Make one of these (Autodesk Fusion 360 design; units mm, degrees)
Autodesk Fusion 360 part; units mm, degrees
sketch "Sketch1" plane through (0, 0, 0) normal (0, 1, 0) x (1, 0, 0)
  line L0 (0, 0) -> (76.2, 0)
  line L1 (76.2, 0) -> (76.2, 266.7)
  line L2 (76.2, 266.7) -> (0, 266.7)
  line L3 (0, 266.7) -> (0, 0)
  constraint horizontal L0
  constraint vertical L1
  constraint horizontal L2
  constraint vertical L3
  constraint coincident L0.start L3.end
extrude "Extrude1" add sketch "Sketch1" along normal blind 6.35
sketch "Sketch2" plane through (0, 6.35, 0) normal (0, 1, 0) x (-1, 0, 0)
  line L0 (0, -266.7) -> (0, 0)
  line L1 (0, 0) -> (-76.2, 0)
  line L2 (-76.2, 0) -> (-76.2, -266.7)
  line L3 (-76.2, -266.7) -> (0, -266.7)
  circle A0 centre (-25.4, -12.7) radius 1.27
  dimension "d3" = 2.54
  measures "d3" diameter of A0
extrude "Extrude2" cut sketch "Sketch2" against normal blind 6.35 contours A0
sketch "Sketch3" plane through (0, 6.35, 0) normal (0, 1, 0) x (-1, 0, 0)
  circle A0 centre (-25.4, -12.7) radius 1.27
  line L0 (0, -266.7) -> (0, 0)
  line L1 (0, 0) -> (-76.2, 0)
  line L2 (-76.2, 0) -> (-76.2, -266.7)
  line L3 (-76.2, -266.7) -> (0, -266.7)
  circle A1 centre (-50.8, -12.7) radius 1.27
  circle A2 centre (-25.4, -254) radius 1.27
  circle A3 centre (-50.8, -254) radius 1.27
  dimension "d6" = 2.54
  dimension "d7" = 2.54
  dimension "d8" = 2.54
  measures "d6" diameter of A1
  measures "d7" diameter of A2
  measures "d8" diameter of A3
extrude "Extrude3" cut sketch "Sketch3" against normal blind 6.35 contours A1 | A2 | A3
sketch "Sketch4" plane through (0, 6.35, 0) normal (0, 1, 0) x (-1, 0, 0)
  circle A0 centre (-50.8, -12.7) radius 1.27
  circle A1 centre (-50.8, -254) radius 1.27
  circle A2 centre (-25.4, -254) radius 1.27
  circle A3 centre (-25.4, -12.7) radius 1.27
  line L0 (0, -266.7) -> (0, 0)
  line L1 (0, 0) -> (-76.2, 0)
  line L2 (-76.2, 0) -> (-76.2, -266.7)
  line L3 (-76.2, -266.7) -> (0, -266.7)
  line L4 (-25.4, -146.05) -> (-50.8, -146.05)
  line L5 (-50.8, -146.05) -> (-50.8, -120.65)
  line L6 (-50.8, -120.65) -> (-25.4, -120.65)
  line L7 (-25.4, -120.65) -> (-25.4, -146.05)
  dimension "d11" = 25.4
  dimension "d12" = 25.4
  constraint horizontal L4
  constraint vertical L5
  constraint horizontal L6
  constraint vertical L7
  measures "d11" distance of L4.start L4.end
  measures "d12" distance of L4.start L6.end
extrude "Extrude4" cut sketch "Sketch4" against normal blind 6.35 contours L4 L5 L6 L7
sketch "Sketch5" plane through (0, 6.35, 0) normal (0, 1, 0) x (-1, 0, 0)
  line L0 (-50.8, -146.05) -> (-50.8, -120.65)
  line L1 (-50.8, -120.65) -> (-25.4, -120.65)
  line L2 (-25.4, -120.65) -> (-25.4, -146.05)
  line L3 (-25.4, -146.05) -> (-50.8, -146.05)
  circle A0 centre (-50.8, -12.7) radius 1.27
  circle A1 centre (-50.8, -254) radius 1.27
  circle A2 centre (-25.4, -254) radius 1.27
  circle A3 centre (-25.4, -12.7) radius 1.27
  line L4 (0, -266.7) -> (0, 0)
  line L5 (0, 0) -> (-76.2, 0)
  line L6 (-76.2, 0) -> (-76.2, -266.7)
  line L7 (-76.2, -266.7) -> (0, -266.7)
  line L8 (-50.8, -146.05) -> (-53.34, -146.05)
  line L9 (-53.34, -146.05) -> (-53.34, -120.65)
  line L10 (-53.34, -120.65) -> (-50.8, -120.65)
  line L11 (-50.8, -120.65) -> (-50.8, -146.05)
  line L12 (-22.86, -148.59) -> (-53.34, -148.59)
  line L13 (-53.34, -148.59) -> (-53.34, -146.05)
  line L14 (-53.34, -146.05) -> (-22.86, -146.05)
  line L15 (-22.86, -146.05) -> (-22.86, -148.59)
  line L16 (-22.86, -146.05) -> (-25.4, -146.05)
  line L17 (-25.4, -146.05) -> (-25.4, -118.11)
  line L18 (-25.4, -118.11) -> (-22.86, -118.11)
  line L19 (-22.86, -118.11) -> (-22.86, -146.05)
  line L20 (-25.4, -118.11) -> (-53.34, -118.11)
  line L21 (-53.34, -118.11) -> (-53.34, -120.65)
  line L22 (-53.34, -120.65) -> (-25.4, -120.65)
  line L23 (-25.4, -120.65) -> (-25.4, -118.11)
  constraint horizontal L8
  constraint vertical L9
  constraint horizontal L10
  constraint vertical L11
  constraint coincident L0.start L3.end
  constraint horizontal L12
  constraint vertical L13
  constraint horizontal L14
  constraint vertical L15
  constraint horizontal L16
  constraint vertical L17
  constraint horizontal L18
  constraint vertical L19
  constraint horizontal L20
  constraint vertical L21
  constraint horizontal L22
  constraint vertical L23
extrude "Extrude5" cut sketch "Sketch5" against normal blind 6.35 contours L0 L8 L9 L10 L11 L14 L22 | L3 L8 L12 L13 L14 L15 L16 | L1 L10 L17 L20 L21 L22 L23 | L2 L14 L16 L17 L18 L19 L23
